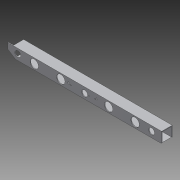
# Autodesk Inventor part: RightMainBeam
Saved by Autodesk Inventor 2013 (Build 170138000, 138)
## iProperties
Created: 2013-02-02
Part Number: RightMainBeam
Material: Aluminum 6061
Document SubType Name: Modeling
Designer: grtstudent
Density: 2.71 g/cm^3
Mass: 1089.63 g
Surface Area: 2589.1 cm^2
Volume: 402.078 cm^3
Author: grtstudent
Autodesk Inventor part; units mm, degrees
ref_plane "YZ Plane" through (0, 0, 0) normal (1, 0, 0) x (0, 1, 0)
ref_plane "XZ Plane" through (0, 0, 0) normal (0, 1, 0) x (-1, 0, 0)
ref_plane "XY Plane" through (0, 0, 0) normal (0, 0, 1) x (1, 0, 0)
sketch "Sketch1" plane through (0, 0, 0) normal (1, 0, 0) x (0, 1, 0)
  line L0 (0, 0) -> (50.8, 0)
  line L1 (50.8, 0) -> (50.8, 50.8)
  line L2 (50.8, 50.8) -> (0, 50.8)
  line L3 (0, 50.8) -> (0, 0)
  line L4 (3.175, 47.625) -> (47.625, 47.625)
  line L5 (47.625, 47.625) -> (47.625, 3.175)
  line L6 (47.625, 3.175) -> (3.175, 3.175)
  line L7 (3.175, 3.175) -> (3.175, 47.625)
  dimension "d0" = 50.8
  dimension "d1" = 3.175
  constraints: 16 end point, 4 parallel, 3 perpendicular, 1 horizontal, 3 other
  measures "d0" distance of L2.end L0.start
  measures "d1" distance between parallel lines of L2 L4
extrude "Extrusion1" add sketch "Sketch1" along normal blind 736.6
sketch "Sketch2" plane through (0, 0, 50.8) normal (0, 0, 1) x (1, 0, 0)
  line L0 (0, 50.8) -> (0, 0) projected
  line L1 (0, 0) -> (736.6, 0) projected
  line L2 (736.6, 50.8) -> (736.6, 0) projected
  line L3 (0, 50.8) -> (736.6, 50.8) projected
  circle A0 centre (48.0624, 26.9875) radius 14.2875
  circle A1 centre (368.3, 23.8125) radius 14.2875
  circle A2 centre (688.5376, 26.9875) radius 14.2875
  line L4 (-35.152, 25.4) -> (810.7598, 25.4) construction
  line L5 (736.6, 3.175) -> (736.6, 0)
  line L6 (736.6, 0) -> (733.425, 0)
  arc A3 (733.425, 0) -> (736.6, 3.175) centre (733.425, 3.175) ccw
  arc A4 (0, 25.4) -> (1.4704, 22.7214) centre (3.175, 25.4) ccw
  arc A5 (36.3954, 0.4964) -> (38.1, 0) centre (38.1, 3.175) ccw
  line L7 (1.4704, 22.7214) -> (36.3954, 0.4964)
  line L8 (0, 25.4) -> (0, 0)
  line L9 (38.1, 0) -> (0, 0)
  line L10 (-134.201, 26.9875) -> (938.3775, 26.9875) construction
  dimension "d4" = 25.4
  dimension "d5" = 23.8125
  dimension "d6" = 320.2534
  dimension "d7" = 320.2534
  dimension "d8" = 368.3
  dimension "d9" = 28.575
  dimension "d10" = 3.175
  dimension "d11" = 3.175
  dimension "d12" = 3.175
  dimension "d13" = 3.175
  dimension "d14" = 38.1
  dimension "d19" = 1.5875
  constraints: 14 end point, 7 point on line, 6 centre point, 6 point on circle, 6 tangent, 3 collinear, 2 equal radius, 2 parallel, 1 midpoint
  measures "d4" distance between parallel lines of L4 L3
  measures "d5" distance from line of L1 A1.centre
  measures "d6" distance of A1.centre A0.centre
  measures "d7" distance of A2.centre A1.centre
  measures "d8" distance from line of L2 A1.centre
  measures "d9" diameter of A0
  measures "d10" distance of L1.end L5.start
  measures "d11" distance of L1.end L6.end
  measures "d12" radius of A4
  measures "d13" radius of A5
  measures "d14" distance from line of L0 A5.centre
  measures "d19" distance between parallel lines of L10 L4
extrude "Extrusion2" cut sketch "Sketch2" against normal blind 50.8 contours A4 L7 A5 L1 L0 | L2 L1 A3 | A0 | A1 | A2
sketch "Sketch3" plane through (736.6, 50.8, 0) normal (0, 0, -1) x (-1, 0, 0)
  line L0 (736.6, 0) -> (711.2, 0)
  line L1 (711.2, 0) -> (711.2, -25.4)
  line L2 (711.2, -25.4) -> (736.6, -25.4)
  line L3 (736.6, -25.4) -> (736.6, 0)
  line L4 (711.2, -25.4) -> (717.8505, -18.7495) construction
  circle A0 centre (713.4451, -23.1549) radius 3.175
  point P0 (736.6, -50.8)
  dimension "d24" = 6.35
  dimension "d17" = 25.4
  dimension "d22" = 45
  constraints: 10 end point, 2 parallel, 2 perpendicular, 1 horizontal, 1 point on line, 3 other
  measures "d17" distance of L0.end L1.end
  measures "d22" angle of L2 L4
extrude "Extrusion3" cut sketch "Sketch3" against normal blind 47.625
sketch "Sketch5" plane through (0, 50.8, 50.8) normal (0, 0, 1) x (1, 0, 0)
  line L0 (0, 0) -> (736.6, 0) projected
  line L1 (0, 0) -> (0, -25.4) projected
  circle A0 centre (368.3, -26.9875) radius 14.2875 projected
  line L2 (-82.8733, -25.4) -> (895.8965, -25.4) construction
  circle A1 centre (127, -25.4) radius 20.32
  circle A2 centre (254, -25.4) radius 20.32
  circle A3 centre (482.6, -25.4) radius 20.32
  circle A4 centre (609.6, -25.4) radius 20.32
  point P0 (0, -50.8)
  dimension "d25" = 25.4
  dimension "d26" = 40.64
  dimension "d27" = 127
  dimension "d28" = 127
  dimension "d29" = 114.3
  dimension "d30" = 114.3
  constraints: 4 centre point, 4 point on line, 3 equal radius, 2 end point, 1 perpendicular
  measures "d25" distance between parallel lines of L0 L2
  measures "d26" diameter of A1
  measures "d27" distance of A2.centre A1.centre
  measures "d28" distance of A4.centre A3.centre
  measures "d29" horizontal distance of A0.centre A2.centre
  measures "d30" horizontal distance of A0.centre A3.centre
extrude "Extrusion4" cut sketch "Sketch5" against normal blind 3.175 contours A1 | A2 | A3 | A4
sketch "Sketch6" plane through (733.425, 0, 0) normal (0, 0, -1) x (-1, 0, 0)
  line L0 (733.425, 25.4) -> (712.5151, 25.4) projected
  circle A0 centre (365.125, 23.8125) radius 14.2875 projected
  line L1 (217.4406, 23.9141) -> (492.0781, 23.9141) construction
  point P0 (733.425, 0)
  point P1 (432.3588, 23.9141)
  point P2 (344.424, 23.9141)
  point P3 (317.0936, 23.9141)
  dimension "d33" = 0.1016
  dimension "d34" = 20.701
  dimension "d35" = 48.0314
  dimension "d36" = 67.2338
  constraints: 3 point on line, 2 end point, 1 parallel
  measures "d33" distance from line of A0.centre L1
  measures "d34" horizontal distance of A0.centre point (344.424, 23.914)
  measures "d35" horizontal distance of A0.centre point (317.094, 23.914)
  measures "d36" distance of point (432.359, 23.914) A0.centre
hole "Hole1" at (301.0662, 23.9141, 0) at (389.001, 23.9141, 0) at (416.3314, 23.9141, 0) direction (0, 0, 1) diameter 7.9756 depth 25.4 tip angle 118
sketch "Sketch7" plane through (733.425, 0, 0) normal (0, 0, -1) x (-1, 0, 0)
  line L0 (733.425, 25.4) -> (712.5151, 25.4) projected
  circle A0 centre (365.125, 23.8125) radius 14.2875 projected
  line L1 (252.4125, 28.8925) -> (487.3625, 28.8925) construction
  point P0 (733.425, 0)
  point P1 (307.5686, 28.8925)
  point P2 (441.8838, 28.8925)
  dimension "d44" = 5.08
  dimension "d45" = 57.5564
  dimension "d46" = 76.7588
  constraints: 2 end point, 2 point on line, 1 parallel
  measures "d44" distance from line of L1 A0.centre
  measures "d45" horizontal distance of A0.centre point (307.569, 28.892)
  measures "d46" horizontal distance of point (441.884, 28.893) A0.centre
hole "Hole2" at (425.8564, 28.8925, 0) at (291.5412, 28.8925, 0) direction (0, 0, 1) diameter 6.35 depth 25.4 tip angle 118
sketch "Sketch8" plane through (0, 50.8, 50.8) normal (0, 0, 1) x (1, 0, 0)
  circle A0 centre (482.6, -25.4) radius 20.32 projected
  circle A1 centre (127, -25.4) radius 20.32 projected
  circle A2 centre (254, -25.4) radius 20.32 projected
  circle A3 centre (609.6, -25.4) radius 20.32 projected
  arc A4 (36.3954, -50.3036) -> (38.1, -50.8) centre (38.1, -47.625) ccw projected
  line L0 (38.1, -50.8) -> (733.425, -50.8) projected
  arc A5 (733.425, -50.8) -> (736.6, -47.625) centre (733.425, -47.625) ccw projected
  line L1 (736.6, 0) -> (736.6, -47.625) projected
  line L2 (0, 0) -> (736.6, 0) projected
  line L3 (0, 0) -> (0, -25.4) projected
  arc A6 (0, -25.4) -> (1.4704, -28.0786) centre (3.175, -25.4) ccw projected
  line L4 (1.4704, -28.0786) -> (36.3954, -50.3036) projected
  circle A7 centre (368.3, -26.9875) radius 14.2875 projected
  circle A8 centre (48.0624, -23.8125) radius 14.2875 projected
  circle A9 centre (688.5376, -23.8125) radius 14.2875 projected
  circle A10 centre (291.5412, -21.9075) radius 3.175 projected
  circle A11 centre (301.0662, -26.8859) radius 3.9878 projected
  circle A12 centre (389.001, -26.8859) radius 3.9878 projected
  circle A13 centre (416.3314, -26.8859) radius 3.9878 projected
  circle A14 centre (425.8564, -21.9075) radius 3.175 projected
  point P0 (0, -50.8)
  constraints: 3 coincident
hole "Hole3" at (301.0662, 23.9141, 50.8) at (389.001, 23.9141, 50.8) at (416.3314, 23.9141, 50.8) direction (0, 0, -1) diameter 4.7625 depth 25.4 tip angle 118
sketch "Sketch9" plane through (0, 50.8, 50.8) normal (0, 0, 1) x (1, 0, 0)
  circle A0 centre (291.5412, -21.9075) radius 3.175 projected
  circle A1 centre (425.8564, -21.9075) radius 3.175 projected
  point P0 (0, -50.8)
  constraints: 2 coincident
hole "Hole4" at (291.5412, 28.8925, 50.8) at (425.8564, 28.8925, 50.8) direction (0, 0, -1) diameter 9.525 depth 25.4 tip angle 118
sketch "Sketch11" plane through (733.425, 0, 0) normal (0, 0, -1) x (-1, 0, 0)
  circle A0 centre (307.5686, 28.8925) radius 3.175 projected
  circle A1 centre (441.8838, 28.8925) radius 3.175 projected
  circle A2 centre (344.424, 23.9141) radius 3.9878 projected
  circle A3 centre (432.3588, 23.9141) radius 3.9878 projected
  circle A4 centre (317.0936, 23.9141) radius 3.9878 projected
  line L0 (708.025, 29.8901) -> (708.025, 50.8) projected
  line L1 (708.025, 50.8) -> (-3.175, 50.8) projected
  line L2 (-3.175, 3.175) -> (-3.175, 50.8) projected
  arc A5 (-3.175, 3.175) -> (0, 0) centre (0, 3.175) ccw projected
  line L3 (695.325, 0) -> (0, 0) projected
  arc A6 (695.325, 0) -> (697.0296, 0.4964) centre (695.325, 3.175) ccw projected
  line L4 (697.0296, 0.4964) -> (731.9546, 22.7214) projected
  arc A7 (731.9546, 22.7214) -> (733.425, 25.4) centre (730.25, 25.4) ccw projected
  line L5 (733.425, 25.4) -> (712.5151, 25.4) projected
  arc A8 (708.025, 29.8901) -> (712.5151, 25.4) centre (710.2701, 27.6451) ccw projected
  circle A9 centre (365.125, 23.8125) radius 14.2875 projected
  circle A10 centre (685.3626, 26.9875) radius 14.2875 projected
  circle A11 centre (44.8874, 26.9875) radius 14.2875 projected
  point P0 (733.425, 0)
sketch "Sketch12" plane through (733.425, 0, 0) normal (0, 0, -1) x (-1, 0, 0)
  circle A0 centre (307.5686, 28.8925) radius 3.175 projected
  circle A1 centre (441.8838, 28.8925) radius 3.175 projected
  circle A2 centre (344.424, 23.9141) radius 3.9878 projected
  circle A3 centre (432.3588, 23.9141) radius 3.9878 projected
  circle A4 centre (317.0936, 23.9141) radius 3.9878 projected
  line L0 (708.025, 29.8901) -> (708.025, 50.8) projected
  line L1 (708.025, 50.8) -> (-3.175, 50.8) projected
  line L2 (-3.175, 3.175) -> (-3.175, 50.8) projected
  arc A5 (-3.175, 3.175) -> (0, 0) centre (0, 3.175) ccw projected
  line L3 (695.325, 0) -> (0, 0) projected
  arc A6 (695.325, 0) -> (697.0296, 0.4964) centre (695.325, 3.175) ccw projected
  line L4 (697.0296, 0.4964) -> (731.9546, 22.7214) projected
  arc A7 (731.9546, 22.7214) -> (733.425, 25.4) centre (730.25, 25.4) ccw projected
  line L5 (733.425, 25.4) -> (712.5151, 25.4) projected
  arc A8 (708.025, 29.8901) -> (712.5151, 25.4) centre (710.2701, 27.6451) ccw projected
  circle A9 centre (365.125, 23.8125) radius 14.2875 projected
  circle A10 centre (685.3626, 26.9875) radius 14.2875 projected
  circle A11 centre (44.8874, 26.9875) radius 14.2875 projected
  line L6 (713.7121, 11.1125) -> (756.5701, 38.3858)
  line L7 (733.425, 25.4) -> (733.425, 4.1402)
  line L8 (695.325, 0) -> (700.957, 0)
  line L9 (713.7121, 11.1125) -> (685.3626, -6.9281)
  line L10 (733.425, 23.6571) -> (740.2433, 12.9426)
  line L11 (696.2496, 0) -> (703.0679, -10.7145)
  line L12 (740.2433, 12.9426) -> (733.425, 12.9426)
  line L13 (703.0679, -10.7145) -> (703.0679, 0)
  line L14 (703.0679, 0) -> (696.2496, 0)
  point P0 (733.425, 0)
  dimension "d69" = 12.7
  dimension "d70" = 12.7
  dimension "d71" = 10.7145
  dimension "d72" = 6.8183
  dimension "d75" = 6.8183
  dimension "d76" = 37.1754
  dimension "d77" = 23.6571
  constraints: 18 end point, 7 point on line, 6 perpendicular, 2 tangent, 1 collinear, 1 parallel
  measures "d69" distance of L10.start L10.end
  measures "d70" distance of L11.start L11.end
  measures "d71" distance from line of L12 L10.start
  measures "d72" distance of L10.end L12.end
  measures "d75" distance of L11.start L13.end
  measures "d76" horizontal distance of L10.start L11.start
  measures "d77" vertical distance of L10.start L11.start
equation "\"d7\" = d6"
equation "\"d11\" = d10"
equation "\"d13\" = d12"
equation "\"d28\" = d27"
equation "\"d30\" = d29"
body "Solid1"
